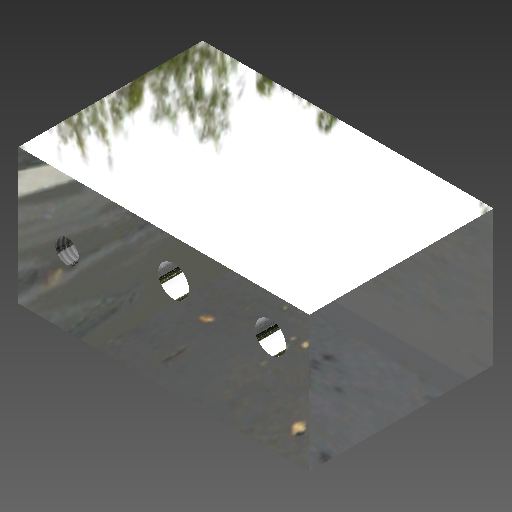
# Autodesk Inventor part: 3d_LM-Welding_Tooling -  Moving Block
Saved by Autodesk Inventor 2018.3 (Build 223284000, 284)
## iProperties
Created: 2026-01-30
Part Number: 3d_LM-Welding_Tooling -  Moving Block
Material: Aluminium 6061-T6
Document SubType Name: Modeling
Designer: aca6
Density: 2.7 g/cm^3
Appearance: N/A - Machined Aluminium
Mass: 20.1118 g
Surface Area: 30.4464 cm^2
Volume: 7.44881 cm^3
Manufacturer-1: {"Name": "Hanstar Technologies Co., Ltd", "PartNumber": "3d_Welding_Tooling -  Moving Block", "Link": ""}
Manufacturer-2: {"Name": "SHENZHEN JINYIHE PROTOTYPE TECHNOLOGIES CO., LTD", "PartNumber": "3d_Welding_Tooling -  Moving Block", "Link": ""}
Manufacturer-3: {"Name": "Shenzhen city Xavier Precision Co., Ltd.", "PartNumber": "3d_Welding_Tooling -  Moving Block", "Link": ""}
Manufacturer-4: {"Name": "", "PartNumber": "", "Link": ""}
Manufacturer-5: {"Name": "", "PartNumber": "", "Link": ""}
Provider-1: {"Name": "", "PartNumber": "", "Link": ""}
Provider-2: {"Name": "", "PartNumber": "", "Link": ""}
Provider-3: {"Name": "", "PartNumber": "", "Link": ""}
Provider-4: {"Name": "", "PartNumber": "", "Link": ""}
Provider-5: {"Name": "", "PartNumber": "", "Link": ""}
Author: aca6
Comments: DIN-ISO-2768-fH
Autodesk Inventor part; units mm, degrees
ref_plane "YZ Plane" through (0, 0, 0) normal (1, 0, 0) x (0, 1, 0)
ref_plane "XZ Plane" through (0, 0, 0) normal (0, 1, 0) x (-1, 0, 0)
ref_plane "XY Plane" through (0, 0, 0) normal (0, 0, 1) x (1, 0, 0)
sketch "Sketch1" plane through (0, 0, 0) normal (0, 0, 1) x (1, 0, 0)
  line L0 (-15, 10.1715) -> (15, 10.1715)
  line L1 (15, 10.1715) -> (15, -10.1715)
  line L2 (15, -10.1715) -> (-15, -10.1715)
  line L3 (-15, -10.1715) -> (-15, 10.1715)
  line L4 (0, 0) -> (0, 4.8999) construction
  line L5 (0, 0) -> (4.2328, 0) construction
  dimension "d2" = 20.343
  dimension "d3" = 30
  constraints: 12 end point, 3 horizontal, 2 parallel, 2 vertical, 1 perpendicular, 4 other
  measures "d2" distance of L2.end L0.start
  measures "d3" distance of L0.start L0.end
extrude "Extrusion1" add sketch "Sketch1" along normal blind 19
sketch "Sketch2" plane through (15, -10.1715, 0) normal (1, 0, 0) x (0, 0, -1)
  line L0 (0, 0) -> (-19, 0) projected
  line L1 (0, 0) -> (-30, 0)
  line L2 (-30, 0) -> (-30, 6.343)
  line L3 (-30, 6.343) -> (0, 6.343)
  line L4 (0, 6.343) -> (0, 0)
  point P0 (0, 10.1715)
  dimension "d4" = 30
  dimension "d5" = 6.343
  constraints: 8 end point, 2 parallel, 1 horizontal, 1 perpendicular
  measures "d4" distance of L2.end L3.end
  measures "d5" distance of L1.end L2.end
extrude "Extrusion2" cut sketch "Sketch2" against normal up to next
sketch "Sketch3" plane through (0, 0, 19) normal (0, 0, 1) x (1, 0, 0)
  line L0 (15, 10.1715) -> (-15, 10.1715) projected
  line L1 (-15, 10.1715) -> (-15, -10.1715) projected
  line L2 (15, -10.1715) -> (15, 10.1715) projected
  point P0 (0, 0)
  point P1 (1, 6.1715)
  point P2 (11, 6.1715)
  dimension "d8" = 4
  dimension "d9" = 4
  dimension "d17" = 16
  dimension "d18" = 4
  measures "d8" distance from line of L0 point (1, 6.172)
  measures "d9" distance from line of L0 point (11, 6.172)
  measures "d17" distance from line of L1 point (1, 6.172)
  measures "d18" distance from line of L2 point (11, 6.172)
hole "Hole1" at (1, 6.1715, 19) at (11, 6.1715, 19) direction (0, 0, -1) diameter 3.2 end through all
sketch "Sketch4" plane through (-15, -10.1715, 19) normal (-1, 0, 0) x (0, 0, 1)
  circle A0 centre (-6.5, 13.5145) radius 2.5 projected
  point P0 (-19, 10.1715)
hole "Hole2" at (-15, 3.343, 12.5) direction (1, 0, 0) diameter 5 depth 10 tip angle 118
sketch "Sketch6" plane through (0, 0, 19) normal (0, 0, 1) x (1, 0, 0)
  line L0 (-15, 0.843) -> (-15, 5.843) projected
  point P0 (0, 0)
  point P1 (-10, 3.343)
  point P2 (-15, 3.343)
  dimension "d26" = 5
  constraints: 1 horizontal alignment, 1 midpoint
  measures "d26" distance from line of L0 point (-10, 3.343)
hole "Hole3" at (-10, 3.343, 19) direction (0, 0, -1) diameter 2.459 depth 6.05 tip angle 118 thread size "M3x0.5" class "6H" standard "ISO Metric profile"
body "Solid1"
